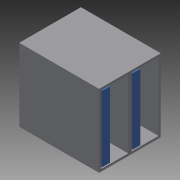
# Autodesk Inventor part: nanopc_t4_usb
Saved by Autodesk Inventor 2013 SP2 (Build 170200200, 200)
## iProperties
Created: 2018-09-03
Part Number: nanopc_t4_usb
Material: Generic
Document SubType Name: Modeling
Designer: alex
Density: 1 g/cm^3
Mass: 1.00072 g
Surface Area: 25.9968 cm^2
Volume: 1.00072 cm^3
Author: alex
Autodesk Inventor part; units mm, degrees
ref_plane "YZ Plane" through (0, 0, 0) normal (1, 0, 0) x (0, 1, 0)
ref_plane "XZ Plane" through (0, 0, 0) normal (0, 1, 0) x (-1, 0, 0)
ref_plane "Work Plane1" through (0, 0.2202, 0) normal (0, 0, 1) x (1, 0, 0)
sketch "Sketch1" plane through (0, 0.2202, 0) normal (0, 0, 1) x (1, 0, 0)
  line L0 (21.9247, 42.5927) -> (36.4247, 42.5927)
  line L1 (36.4247, 42.5927) -> (36.4247, 36.8927)
  line L2 (36.4247, 36.8927) -> (21.9247, 36.8927)
  line L3 (21.9247, 36.8927) -> (21.9247, 42.5927)
  point P0 (0, -0.2202)
  dimension "d0" = 14.5
  dimension "d2" = 5.7
  constraints: 8 end point, 2 parallel, 1 horizontal, 1 perpendicular
  measures "d0" distance of L1.end L2.end
  measures "d2" distance of L0.end L1.end
extrude "Extrusion1" add sketch "Sketch1" along normal blind 13.2
sketch "Sketch2" plane through (36.4247, 37.1129, 0) normal (1, 0, 0) x (0, 0, -1)
  line L0 (0, 5.7) -> (0, 0) projected
  line L1 (0, 5.7) -> (-13.2, 5.7) projected
  line L2 (-13.2, 0) -> (-13.2, 5.7) projected
  line L3 (0, 0) -> (-13.2, 0) projected
  line L4 (-12.8, 5.3) -> (-0.4, 5.3)
  line L5 (-0.4, 5.3) -> (-0.4, 0.4)
  line L6 (-0.4, 0.4) -> (-12.8, 0.4)
  line L7 (-12.8, 0.4) -> (-12.8, 5.3)
  point P0 (0, -37.1129)
  dimension "d5" = 0.4
  constraints: 8 end point, 3 other
  measures "d5" distance between parallel lines of L1 L4
extrude "Extrusion2" cut sketch "Sketch2" against normal blind 13 contours L4 L5 L6 L7
sketch "Sketch3" plane through (23.4247, 37.1129, 0) normal (1, 0, 0) x (0, 0, -1)
  line L0 (-12.8, 0.4) -> (-12.8, 5.3) projected
  line L1 (-0.4, 0.4) -> (-12.8, 0.4) projected
  line L2 (-0.4, 5.3) -> (-0.4, 0.4) projected
  line L3 (-12.6, 2) -> (-0.6, 2)
  line L4 (-0.6, 2) -> (-0.6, 0.6)
  line L5 (-0.6, 0.6) -> (-12.6, 0.6)
  line L6 (-12.6, 0.6) -> (-12.6, 2)
  point P0 (0, -37.1129)
  dimension "d8" = 0.2
  dimension "d9" = 0.2
  dimension "d10" = 0.2
  dimension "d11" = 1.4
  constraints: 8 end point, 2 parallel, 1 horizontal, 1 perpendicular
  measures "d8" distance between parallel lines of L1 L5
  measures "d9" distance between parallel lines of L0 L6
  measures "d10" distance between parallel lines of L2 L4
  measures "d11" distance of L5.end L3.start
extrude "Extrusion3" add sketch "Sketch3" along normal blind 13
pattern_linear "Rectangular Pattern1" count 2 spacing 5.5 along (0, 1, 0) of "Extrusion1", "Extrusion3", "Extrusion2"
body "Solid1"
